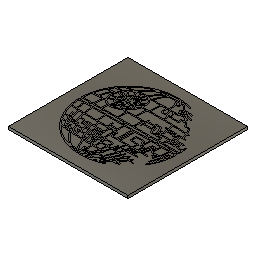
Death Star display v8 (Autodesk Fusion 360 archive; units mm, degrees)
design "Death Star display" references "autodesk 3ax table head yxz"
Autodesk Fusion 360 part; units mm, degrees
(part 1 of 5)
sketch "Sketch1" plane through (0, 0, 0) normal (0, 0, 1) x (1, 0, 0)
  spline S0 degree 3 poles (-1.6299, -34.337) (-1.7839, -34.323) (-2.351, -34.2778) (-2.89, -34.2364) knots 0 0 0 0 1 1 1 1
  spline S1 degree 3 poles (-2.89, -34.2364) (-5.9502, -34.0018) (-9.4769, -33.1887) (-12.4456, -32.0334) knots 0 0 0 0 1 1 1 1
  spline S2 degree 3 poles (-12.4456, -32.0334) (-13.5279, -31.6122) (-13.855, -31.4671) (-15.2108, -30.8071) knots 0 0 0 0 1 1 1 1
  spline S3 degree 3 poles (-15.2108, -30.8071) (-22.0231, -27.4905) (-27.7431, -21.7969) (-31.0912, -15.0001) knots 0 0 0 0 1 1 1 1
  spline S4 degree 3 poles (-31.0912, -15.0001) (-33.1398, -10.8414) (-34.2254, -6.8844) (-34.6063, -2.1874) knots 0 0 0 0 1 1 1 1
  line L0 (-34.6063, -2.1874) -> (-34.7219, -0.7625)
  line L1 (-34.7219, -0.7625) -> (-34.4344, -0.4696)
  line L2 (-34.4344, -0.4696) -> (-34.1469, -0.1767)
  line L3 (-34.1469, -0.1767) -> (-34.1469, 0.483)
  line L4 (-34.1469, 0.483) -> (-34.1469, 1.1428)
  line L5 (-34.1469, 1.1428) -> (-34.4351, 1.4363)
  line L6 (-34.4351, 1.4363) -> (-34.7232, 1.7299)
  line L7 (-34.7232, 1.7299) -> (-34.6057, 3.1541)
  spline S5 degree 3 poles (-34.6057, 3.1541) (-33.9079, 11.6096) (-30.3961, 19.2356) (-24.4881, 25.1245) knots 0 0 0 0 1 1 1 1
  spline S6 degree 3 poles (-24.4881, 25.1245) (-18.2485, 31.3441) (-10.2507, 34.8631) (-1.4199, 35.2745) knots 0 0 0 0 1 1 1 1
  spline S7 degree 3 poles (-1.4199, 35.2745) (2.3869, 35.4519) (6.2534, 34.994) (9.9208, 33.9317) knots 0 0 0 0 1 1 1 1
  spline S8 degree 3 poles (9.9208, 33.9317) (10.9671, 33.6286) (11.0739, 33.5871) (11.2449, 33.416) knots 0 0 0 0 1 1 1 1
  spline S9 degree 3 poles (11.2449, 33.416) (11.3437, 33.3172) (11.3441, 33.2853) (11.2485, 33.1006) knots 0 0 0 0 1 1 1 1
  spline S10 degree 3 poles (11.2485, 33.1006) (11.1766, 32.9614) (11.089, 32.895) (10.9772, 32.895) knots 0 0 0 0 1 1 1 1
  spline S11 degree 3 poles (10.9772, 32.895) (10.8864, 32.895) (10.3281, 33.0339) (9.7364, 33.2037) knots 0 0 0 0 1 1 1 1
  spline S12 degree 3 poles (9.7364, 33.2037) (8.2848, 33.6202) (6.6384, 33.9815) (5.2556, 34.1871) knots 0 0 0 0 1 1 1 1
  spline S13 degree 3 poles (5.2556, 34.1871) (4.2003, 34.3439) (4.1036, 34.3483) (4.0229, 34.2428) knots 0 0 0 0 1 1 1 1
  spline S14 degree 3 poles (4.0229, 34.2428) (3.8864, 34.0642) (3.9187, 33.9997) (4.2949, 33.7001) knots 0 0 0 0 1 1 1 1
  spline S15 degree 3 poles (4.2949, 33.7001) (5.0546, 33.0949) (4.9616, 33.1289) (6.0085, 33.0734) knots 0 0 0 0 1 1 1 1
  spline S16 degree 3 poles (6.0085, 33.0734) (6.537, 33.0454) (7.0379, 32.9965) (7.1215, 32.9647) knots 0 0 0 0 1 1 1 1
  spline S17 degree 3 poles (7.1215, 32.9647) (7.3715, 32.8696) (8.6397, 31.827) (9.4234, 31.0722) knots 0 0 0 0 1 1 1 1
  line L8 (9.4234, 31.0722) -> (10.156, 30.3666)
  line L9 (10.156, 30.3666) -> (11.0184, 30.3026)
  spline S18 degree 3 poles (11.0184, 30.3026) (12.8168, 30.1691) (15.6071, 29.7574) (16.0637, 29.5581) knots 0 0 0 0 1 1 1 1
  spline S19 degree 3 poles (16.0637, 29.5581) (16.3282, 29.4427) (16.3625, 29.3626) (16.2798, 29.0535) knots 0 0 0 0 1 1 1 1
  spline S20 degree 3 poles (16.2798, 29.0535) (16.2375, 28.8956) (16.214, 28.8893) (15.8082, 28.9275) knots 0 0 0 0 1 1 1 1
  spline S21 degree 3 poles (15.8082, 28.9275) (15.5733, 28.9497) (15.1291, 29.0129) (14.8211, 29.0681) knots 0 0 0 0 1 1 1 1
  spline S22 degree 3 poles (14.8211, 29.0681) (13.6561, 29.2768) (13.6729, 29.2766) (13.5839, 29.0812) knots 0 0 0 0 1 1 1 1
  spline S23 degree 3 poles (13.5839, 29.0812) (13.5104, 28.9199) (13.5347, 28.8729) (13.8828, 28.5027) knots 0 0 0 0 1 1 1 1
  spline S24 degree 3 poles (13.8828, 28.5027) (14.0912, 28.2811) (14.3876, 27.9481) (14.5414, 27.7628) knots 0 0 0 0 1 1 1 1
  line L10 (14.5414, 27.7628) -> (14.8211, 27.4259)
  line L11 (14.8211, 27.4259) -> (15.5806, 27.3262)
  spline S25 degree 3 poles (15.5806, 27.3262) (17.4175, 27.0852) (18.6937, 26.7735) (18.9731, 26.4976) knots 0 0 0 0 1 1 1 1
  spline S26 degree 3 poles (18.9731, 26.4976) (19.0983, 26.3741) (19.1239, 26.2944) (19.0866, 26.1456) knots 0 0 0 0 1 1 1 1
  spline S27 degree 3 poles (19.0866, 26.1456) (19.0601, 26.0398) (18.9925, 25.9357) (18.9365, 25.9142) knots 0 0 0 0 1 1 1 1
  spline S28 degree 3 poles (18.9365, 25.9142) (18.8805, 25.8927) (18.4829, 25.9714) (18.053, 26.0889) knots 0 0 0 0 1 1 1 1
  spline S29 degree 3 poles (18.053, 26.0889) (16.8455, 26.4192) (15.9994, 26.5611) (15.8713, 26.4547) knots 0 0 0 0 1 1 1 1
  spline S30 degree 3 poles (15.8713, 26.4547) (15.7138, 26.324) (15.7436, 26.1435) (15.9612, 25.9106) knots 0 0 0 0 1 1 1 1
  spline S31 degree 3 poles (15.9612, 25.9106) (16.1292, 25.7307) (16.2251, 25.6949) (16.6531, 25.6519) knots 0 0 0 0 1 1 1 1
  spline S32 degree 3 poles (16.6531, 25.6519) (17.2658, 25.5904) (17.5932, 25.4158) (17.5357, 25.1814) knots 0 0 0 0 1 1 1 1
  spline S33 degree 3 poles (17.5357, 25.1814) (17.4779, 24.9455) (17.3792, 24.8445) (17.2067, 24.8445) knots 0 0 0 0 1 1 1 1
  spline S34 degree 3 poles (17.2067, 24.8445) (17.0335, 24.8445) (16.8862, 24.7229) (16.8862, 24.5799) knots 0 0 0 0 1 1 1 1
  spline S35 degree 3 poles (16.8862, 24.5799) (16.8862, 24.5267) (16.9924, 24.3204) (17.1221, 24.1213) knots 0 0 0 0 1 1 1 1
  spline S36 degree 3 poles (17.1221, 24.1213) (17.2518, 23.9223) (17.443, 23.6113) (17.5469, 23.4301) knots 0 0 0 0 1 1 1 1
  spline S37 degree 3 poles (17.5469, 23.4301) (17.7574, 23.0631) (17.7742, 23.055) (18.4569, 22.9881) knots 0 0 0 0 1 1 1 1
  spline S38 degree 3 poles (18.4569, 22.9881) (18.724, 22.9619) (19.0145, 22.8933) (19.1025, 22.8357) knots 0 0 0 0 1 1 1 1
  spline S39 degree 3 poles (19.1025, 22.8357) (19.2689, 22.7266) (19.8565, 21.8786) (20.241, 21.1925) knots 0 0 0 0 1 1 1 1
  spline S40 degree 3 poles (20.241, 21.1925) (20.3633, 20.9742) (20.5012, 20.7648) (20.5474, 20.7272) knots 0 0 0 0 1 1 1 1
  spline S41 degree 3 poles (20.5474, 20.7272) (20.5936, 20.6895) (21.2844, 20.6109) (22.0824, 20.5524) knots 0 0 0 0 1 1 1 1
  spline S42 degree 3 poles (22.0824, 20.5524) (23.3363, 20.4606) (23.5611, 20.4264) (23.738, 20.3004) knots 0 0 0 0 1 1 1 1
  spline S43 degree 3 poles (23.738, 20.3004) (23.8876, 20.1939) (24.1714, 19.6967) (24.7902, 18.4568) knots 0 0 0 0 1 1 1 1
  spline S44 degree 3 poles (24.7902, 18.4568) (25.2563, 17.523) (25.6374, 16.7208) (25.6372, 16.674) knots 0 0 0 0 1 1 1 1
  spline S45 degree 3 poles (25.6372, 16.674) (25.6364, 16.5295) (25.857, 16.4643) (26.5118, 16.4154) knots 0 0 0 0 1 1 1 1
  spline S46 degree 3 poles (26.5118, 16.4154) (26.8583, 16.3895) (27.2442, 16.3357) (27.3694, 16.2957) knots 0 0 0 0 1 1 1 1
  spline S47 degree 3 poles (27.3694, 16.2957) (27.5664, 16.2329) (27.5969, 16.1917) (27.5969, 15.9883) knots 0 0 0 0 1 1 1 1
  spline S48 degree 3 poles (27.5969, 15.9883) (27.5969, 15.698) (27.468, 15.6443) (26.8199, 15.6645) knots 0 0 0 0 1 1 1 1
  spline S49 degree 3 poles (26.8199, 15.6645) (26.2136, 15.6833) (26.1253, 15.5947) (26.2847, 15.1273) knots 0 0 0 0 1 1 1 1
  spline S50 degree 3 poles (26.2847, 15.1273) (26.3463, 14.9467) (26.5579, 14.3264) (26.7551, 13.7488) knots 0 0 0 0 1 1 1 1
  spline S51 degree 3 poles (26.7551, 13.7488) (26.9522, 13.1713) (27.1653, 12.6594) (27.2286, 12.6113) knots 0 0 0 0 1 1 1 1
  spline S52 degree 3 poles (27.2286, 12.6113) (27.3005, 12.5565) (27.5755, 12.5238) (27.9625, 12.5238) knots 0 0 0 0 1 1 1 1
  spline S53 degree 3 poles (27.9625, 12.5238) (28.7632, 12.5238) (29.067, 12.4088) (29.067, 12.1058) knots 0 0 0 0 1 1 1 1
  spline S54 degree 3 poles (29.067, 12.1058) (29.067, 11.7499) (28.92, 11.7252) (27.3051, 11.8106) knots 0 0 0 0 1 1 1 1
  spline S55 degree 3 poles (27.3051, 11.8106) (26.0171, 11.8787) (25.8721, 11.875) (25.7564, 11.7703) knots 0 0 0 0 1 1 1 1
  spline S56 degree 3 poles (25.7564, 11.7703) (25.6664, 11.6888) (25.6422, 11.6024) (25.6741, 11.4768) knots 0 0 0 0 1 1 1 1
  spline S57 degree 3 poles (25.6741, 11.4768) (25.8258, 10.8804) (26.1968, 9.1892) (26.1968, 9.094) knots 0 0 0 0 1 1 1 1
  spline S58 degree 3 poles (26.1968, 9.094) (26.1968, 9.0315) (26.2378, 8.9243) (26.2878, 8.8558) knots 0 0 0 0 1 1 1 1
  spline S59 degree 3 poles (26.2878, 8.8558) (26.397, 8.7065) (26.4181, 8.7047) (29.347, 8.5979) knots 0 0 0 0 1 1 1 1
  spline S60 degree 3 poles (29.347, 8.5979) (31.7762, 8.5093) (31.9372, 8.4796) (31.9372, 8.1202) knots 0 0 0 0 1 1 1 1
  spline S61 degree 3 poles (31.9372, 8.1202) (31.9372, 7.8265) (31.6603, 7.7329) (30.9701, 7.7931) knots 0 0 0 0 1 1 1 1
  spline S62 degree 3 poles (30.9701, 7.7931) (30.4875, 7.8352) (30.4115, 7.8254) (30.3047, 7.7074) knots 0 0 0 0 1 1 1 1
  spline S63 degree 3 poles (30.3047, 7.7074) (30.1903, 7.5811) (30.1932, 7.5183) (30.3606, 6.4987) knots 0 0 0 0 1 1 1 1
  spline S64 degree 3 poles (30.3606, 6.4987) (30.4577, 5.9071) (30.5371, 5.3334) (30.5371, 5.2236) knots 0 0 0 0 1 1 1 1
  spline S65 degree 3 poles (30.5371, 5.2236) (30.5371, 4.7238) (30.5851, 4.7101) (32.5383, 4.6524) knots 0 0 0 0 1 1 1 1
  line L12 (32.5383, 4.6524) -> (33.8045, 4.6149)
  line L13 (33.8045, 4.6149) -> (33.8905, 4.7757)
  spline S66 degree 3 poles (33.8905, 4.7757) (33.9606, 4.9066) (33.9499, 5.1007) (33.8326, 5.8222) knots 0 0 0 0 1 1 1 1
  spline S67 degree 3 poles (33.8326, 5.8222) (33.6677, 6.8367) (33.6971, 7.0284) (34.025, 7.0765) knots 0 0 0 0 1 1 1 1
  spline S68 degree 3 poles (34.025, 7.0765) (34.3629, 7.1261) (34.4398, 6.9157) (34.6693, 5.3133) knots 0 0 0 0 1 1 1 1
  spline S69 degree 3 poles (34.6693, 5.3133) (34.7859, 4.4989) (34.9467, 2.6691) (34.9471, 2.1532) knots 0 0 0 0 1 1 1 1
  spline S70 degree 3 poles (34.9471, 2.1532) (34.9473, 1.7163) (34.9311, 1.6686) (34.6759, 1.3598) knots 0 0 0 0 1 1 1 1
  spline S71 degree 3 poles (34.6759, 1.3598) (34.4089, 1.0367) (34.4046, 1.0223) (34.4134, 0.4812) knots 0 0 0 0 1 1 1 1
  spline S72 degree 3 poles (34.4134, 0.4812) (34.4219, -0.0405) (34.4358, -0.0867) (34.6848, -0.4131) knots 0 0 0 0 1 1 1 1
  spline S73 degree 3 poles (34.6848, -0.4131) (34.925, -0.728) (34.9473, -0.7954) (34.9471, -1.2047) knots 0 0 0 0 1 1 1 1
  spline S74 degree 3 poles (34.9471, -1.2047) (34.9465, -1.8462) (34.7588, -3.799) (34.5982, -4.8304) knots 0 0 0 0 1 1 1 1
  spline S75 degree 3 poles (34.5982, -4.8304) (34.0278, -8.4945) (32.9754, -11.7968) (31.3273, -15.0929) knots 0 0 0 0 1 1 1 1
  spline S76 degree 3 poles (31.3273, -15.0929) (30.3393, -17.0691) (30.1369, -17.336) (29.7956, -17.1124) knots 0 0 0 0 1 1 1 1
  spline S77 degree 3 poles (29.7956, -17.1124) (29.6431, -17.0125) (29.6224, -16.9596) (29.6593, -16.763) knots 0 0 0 0 1 1 1 1
  spline S78 degree 3 poles (29.6593, -16.763) (29.6832, -16.6356) (29.815, -16.3337) (29.9521, -16.0922) knots 0 0 0 0 1 1 1 1
  spline S79 degree 3 poles (29.9521, -16.0922) (30.3995, -15.3042) (31.0971, -13.8729) (31.0971, -13.7429) knots 0 0 0 0 1 1 1 1
  spline S80 degree 3 poles (31.0971, -13.7429) (31.0971, -13.5327) (30.9653, -13.4645) (30.6197, -13.4961) knots 0 0 0 0 1 1 1 1
  spline S81 degree 3 poles (30.6197, -13.4961) (30.0164, -13.5513) (29.9895, -13.5672) (29.7731, -13.9958) knots 0 0 0 0 1 1 1 1
  spline S82 degree 3 poles (29.7731, -13.9958) (29.5066, -14.5239) (29.4404, -14.5729) (29.1561, -14.4536) knots 0 0 0 0 1 1 1 1
  spline S83 degree 3 poles (29.1561, -14.4536) (28.9511, -14.3676) (28.9342, -14.3378) (28.9727, -14.1309) knots 0 0 0 0 1 1 1 1
  spline S84 degree 3 poles (28.9727, -14.1309) (28.9961, -14.0055) (29.2122, -13.3988) (29.453, -12.7828) knots 0 0 0 0 1 1 1 1
  spline S85 degree 3 poles (29.453, -12.7828) (29.985, -11.4215) (30.4454, -10.0193) (30.7741, -8.7592) knots 0 0 0 0 1 1 1 1
  spline S86 degree 3 poles (30.7741, -8.7592) (31.0871, -7.5589) (31.0954, -7.5736) (30.1326, -7.62) knots 0 0 0 0 1 1 1 1
  spline S87 degree 3 poles (30.1326, -7.62) (29.6266, -7.6443) (29.423, -7.6822) (29.3388, -7.7676) knots 0 0 0 0 1 1 1 1
  spline S88 degree 3 poles (29.3388, -7.7676) (29.2726, -7.8348) (29.117, -8.377) (28.9642, -9.0726) knots 0 0 0 0 1 1 1 1
  spline S89 degree 3 poles (28.9642, -9.0726) (28.549, -10.9622) (28.4593, -11.1542) (28.0627, -11.0023) knots 0 0 0 0 1 1 1 1
  spline S90 degree 3 poles (28.0627, -11.0023) (27.8758, -10.9308) (27.8653, -10.9055) (27.8924, -10.5944) knots 0 0 0 0 1 1 1 1
  spline S91 degree 3 poles (27.8924, -10.5944) (27.9083, -10.4119) (28.0415, -9.7353) (28.1884, -9.0909) knots 0 0 0 0 1 1 1 1
  spline S92 degree 3 poles (28.1884, -9.0909) (28.4059, -8.1361) (28.4391, -7.8995) (28.3676, -7.8133) knots 0 0 0 0 1 1 1 1
  spline S93 degree 3 poles (28.3676, -7.8133) (28.2583, -7.6816) (27.674, -7.6707) (27.5011, -7.7971) knots 0 0 0 0 1 1 1 1
  spline S94 degree 3 poles (27.5011, -7.7971) (27.4276, -7.8508) (27.328, -8.1099) (27.2522, -8.4446) knots 0 0 0 0 1 1 1 1
  spline S95 degree 3 poles (27.2522, -8.4446) (27.0519, -9.3288) (26.9738, -9.5736) (26.8383, -9.7409) knots 0 0 0 0 1 1 1 1
  spline S96 degree 3 poles (26.8383, -9.7409) (26.7304, -9.8742) (26.681, -9.8874) (26.5067, -9.8297) knots 0 0 0 0 1 1 1 1
  spline S97 degree 3 poles (26.5067, -9.8297) (26.2354, -9.7398) (26.2176, -9.5474) (26.4066, -8.7426) knots 0 0 0 0 1 1 1 1
  spline S98 degree 3 poles (26.4066, -8.7426) (26.4889, -8.3918) (26.5378, -8.0312) (26.5152, -7.9412) knots 0 0 0 0 1 1 1 1
  spline S99 degree 3 poles (26.5152, -7.9412) (26.4743, -7.7779) (26.4711, -7.7775) (25.3255, -7.7775) knots 0 0 0 0 1 1 1 1
  line L14 (25.3255, -7.7775) -> (24.1769, -7.7775)
  line L15 (24.1769, -7.7775) -> (23.9618, -7.5165)
  spline S100 degree 3 poles (23.9618, -7.5165) (23.8435, -7.373) (23.7467, -7.2008) (23.7467, -7.134) knots 0 0 0 0 1 1 1 1
  spline S101 degree 3 poles (23.7467, -7.134) (23.7467, -6.867) (23.0285, -6.7555) (22.8186, -6.9899) knots 0 0 0 0 1 1 1 1
  spline S102 degree 3 poles (22.8186, -6.9899) (22.7547, -7.0613) (22.6474, -7.4785) (22.5614, -7.9898) knots 0 0 0 0 1 1 1 1
  spline S103 degree 3 poles (22.5614, -7.9898) (22.4803, -8.4724) (22.3249, -9.3018) (22.216, -9.833) knots 0 0 0 0 1 1 1 1
  spline S104 degree 3 poles (22.216, -9.833) (21.9451, -11.1548) (21.8426, -11.0705) (23.6417, -11.0042) knots 0 0 0 0 1 1 1 1
  spline S105 degree 3 poles (23.6417, -11.0042) (25.2698, -10.9442) (25.4268, -10.9717) (25.4268, -11.3171) knots 0 0 0 0 1 1 1 1
  spline S106 degree 3 poles (25.4268, -11.3171) (25.4268, -11.4801) (25.3842, -11.5756) (25.2885, -11.6268) knots 0 0 0 0 1 1 1 1
  spline S107 degree 3 poles (25.2885, -11.6268) (25.1384, -11.7072) (22.5954, -11.8346) (21.104, -11.8366) knots 0 0 0 0 1 1 1 1
  spline S108 degree 3 poles (21.104, -11.8366) (20.2707, -11.8376) (20.1622, -11.852) (20.0364, -11.9778) knots 0 0 0 0 1 1 1 1
  spline S109 degree 3 poles (20.0364, -11.9778) (19.9594, -12.0548) (19.8964, -12.1629) (19.8964, -12.218) knots 0 0 0 0 1 1 1 1
  spline S110 degree 3 poles (19.8964, -12.218) (19.8964, -12.3489) (19.354, -14.4146) (19.2646, -14.6244) knots 0 0 0 0 1 1 1 1
  spline S111 degree 3 poles (19.2646, -14.6244) (19.2176, -14.7346) (19.2207, -14.8326) (19.2743, -14.9328) knots 0 0 0 0 1 1 1 1
  spline S112 degree 3 poles (19.2743, -14.9328) (19.3513, -15.0766) (19.3806, -15.0787) (20.7064, -15.0343) knots 0 0 0 0 1 1 1 1
  spline S113 degree 3 poles (20.7064, -15.0343) (22.2673, -14.982) (22.4166, -15.0102) (22.4166, -15.3572) knots 0 0 0 0 1 1 1 1
  spline S114 degree 3 poles (22.4166, -15.3572) (22.4166, -15.5566) (22.384, -15.6013) (22.1891, -15.67) knots 0 0 0 0 1 1 1 1
  spline S115 degree 3 poles (22.1891, -15.67) (21.9751, -15.7454) (20.071, -15.8452) (17.2012, -15.9315) knots 0 0 0 0 1 1 1 1
  spline S116 degree 3 poles (17.2012, -15.9315) (16.5082, -15.9524) (15.4904, -15.9888) (14.9395, -16.0124) knots 0 0 0 0 1 1 1 1
  spline S117 degree 3 poles (14.9395, -16.0124) (13.7776, -16.0622) (13.8181, -16.0365) (13.6328, -16.8431) knots 0 0 0 0 1 1 1 1
  spline S118 degree 3 poles (13.6328, -16.8431) (13.5709, -17.1126) (13.4084, -17.7232) (13.2718, -18.1999) knots 0 0 0 0 1 1 1 1
  spline S119 degree 3 poles (13.2718, -18.1999) (12.9494, -19.3249) (12.9251, -19.2946) (14.2001, -19.3546) knots 0 0 0 0 1 1 1 1
  spline S120 degree 3 poles (14.2001, -19.3546) (14.9341, -19.3892) (15.1353, -19.3786) (15.199, -19.3018) knots 0 0 0 0 1 1 1 1
  spline S121 degree 3 poles (15.199, -19.3018) (15.2428, -19.249) (15.3974, -18.8946) (15.5424, -18.5144) knots 0 0 0 0 1 1 1 1
  spline S122 degree 3 poles (15.5424, -18.5144) (15.8798, -17.6298) (15.9501, -17.5081) (16.1232, -17.5081) knots 0 0 0 0 1 1 1 1
  spline S123 degree 3 poles (16.1232, -17.5081) (16.5865, -17.5081) (16.6391, -17.7921) (16.3262, -18.6046) knots 0 0 0 0 1 1 1 1
  spline S124 degree 3 poles (16.3262, -18.6046) (16.2107, -18.9046) (16.1162, -19.1852) (16.1162, -19.2283) knots 0 0 0 0 1 1 1 1
  spline S125 degree 3 poles (16.1162, -19.2283) (16.1162, -19.4449) (16.371, -19.5217) (17.2488, -19.5698) knots 0 0 0 0 1 1 1 1
  spline S126 degree 3 poles (17.2488, -19.5698) (18.2871, -19.6267) (18.1667, -19.7081) (18.6413, -18.6282) knots 0 0 0 0 1 1 1 1
  spline S127 degree 3 poles (18.6413, -18.6282) (18.802, -18.2624) (18.9969, -17.8936) (19.0743, -17.8087) knots 0 0 0 0 1 1 1 1
  spline S128 degree 3 poles (19.0743, -17.8087) (19.2055, -17.6647) (19.2287, -17.6612) (19.4157, -17.7579) knots 0 0 0 0 1 1 1 1
  spline S129 degree 3 poles (19.4157, -17.7579) (19.693, -17.9013) (19.6812, -18.1981) (19.3714, -18.878) knots 0 0 0 0 1 1 1 1
  spline S130 degree 3 poles (19.3714, -18.878) (19.0989, -19.476) (19.0839, -19.5558) (19.2222, -19.6706) knots 0 0 0 0 1 1 1 1
  spline S131 degree 3 poles (19.2222, -19.6706) (19.3492, -19.776) (20.8787, -19.962) (21.0157, -19.8886) knots 0 0 0 0 1 1 1 1
  spline S132 degree 3 poles (21.0157, -19.8886) (21.0746, -19.8571) (21.2695, -19.5679) (21.4487, -19.246) knots 0 0 0 0 1 1 1 1
  spline S133 degree 3 poles (21.4487, -19.246) (21.628, -18.924) (21.8425, -18.5992) (21.9254, -18.5242) knots 0 0 0 0 1 1 1 1
  spline S134 degree 3 poles (21.9254, -18.5242) (22.0636, -18.3991) (22.0917, -18.3965) (22.2633, -18.4929) knots 0 0 0 0 1 1 1 1
  spline S135 degree 3 poles (22.2633, -18.4929) (22.5344, -18.645) (22.5308, -18.7917) (22.2419, -19.3763) knots 0 0 0 0 1 1 1 1
  spline S136 degree 3 poles (22.2419, -19.3763) (22.0019, -19.8618) (21.9919, -19.9071) (22.0975, -20.0238) knots 0 0 0 0 1 1 1 1
  spline S137 degree 3 poles (22.0975, -20.0238) (22.1651, -20.0985) (22.359, -20.1668) (22.5763, -20.1925) knots 0 0 0 0 1 1 1 1
  spline S138 degree 3 poles (22.5763, -20.1925) (23.2927, -20.2773) (24.4852, -20.5929) (24.6804, -20.7493) knots 0 0 0 0 1 1 1 1
  spline S139 degree 3 poles (24.6804, -20.7493) (24.8574, -20.8912) (24.8662, -20.9211) (24.7927, -21.1308) knots 0 0 0 0 1 1 1 1
  spline S140 degree 3 poles (24.7927, -21.1308) (24.7255, -21.3228) (24.6786, -21.3582) (24.4923, -21.3576) knots 0 0 0 0 1 1 1 1
  spline S141 degree 3 poles (24.4923, -21.3576) (24.371, -21.357) (24.1142, -21.3087) (23.9216, -21.2499) knots 0 0 0 0 1 1 1 1
  spline S142 degree 3 poles (23.9216, -21.2499) (23.4341, -21.1009) (21.6392, -20.791) (21.5088, -20.8333) knots 0 0 0 0 1 1 1 1
  spline S143 degree 3 poles (21.5088, -20.8333) (21.4498, -20.8524) (21.1691, -21.2383) (20.885, -21.6907) knots 0 0 0 0 1 1 1 1
  spline S144 degree 3 poles (20.885, -21.6907) (20.2516, -22.6996) (19.7939, -23.3575) (19.1863, -24.1324) knots 0 0 0 0 1 1 1 1
  spline S145 degree 3 poles (19.1863, -24.1324) (18.852, -24.5587) (18.7317, -24.7655) (18.7585, -24.8679) knots 0 0 0 0 1 1 1 1
  spline S146 degree 3 poles (18.7585, -24.8679) (18.779, -24.9463) (18.8308, -25.0205) (18.8735, -25.0329) knots 0 0 0 0 1 1 1 1
  spline S147 degree 3 poles (18.8735, -25.0329) (20.1001, -25.3867) (20.4228, -25.6622) (20.2083, -26.1724) knots 0 0 0 0 1 1 1 1
  spline S148 degree 3 poles (20.2083, -26.1724) (20.085, -26.4656) (19.6172, -26.6956) (18.776, -26.8766) knots 0 0 0 0 1 1 1 1
  spline S149 degree 3 poles (18.776, -26.8766) (18.185, -27.0038) (16.7415, -27.2387) (16.551, -27.2387) knots 0 0 0 0 1 1 1 1
  spline S150 degree 3 poles (16.551, -27.2387) (16.5113, -27.2387) (16.1688, -27.5252) (15.7899, -27.8754) knots 0 0 0 0 1 1 1 1
  spline S151 degree 3 poles (15.7899, -27.8754) (14.7516, -28.8352) (13.5283, -29.7985) (12.4388, -30.5143) knots 0 0 0 0 1 1 1 1
  spline S152 degree 3 poles (12.4388, -30.5143) (10.9769, -31.4747) (10.9358, -31.5033) (10.9358, -31.5615) knots 0 0 0 0 1 1 1 1
  spline S153 degree 3 poles (10.9358, -31.5615) (10.9358, -31.5911) (10.9962, -31.653) (11.07, -31.6991) knots 0 0 0 0 1 1 1 1
  spline S154 degree 3 poles (11.07, -31.6991) (11.1827, -31.7694) (11.3767, -31.7174) (12.2776, -31.375) knots 0 0 0 0 1 1 1 1
  spline S155 degree 3 poles (12.2776, -31.375) (12.868, -31.1507) (13.5991, -30.8528) (13.9023, -30.713) knots 0 0 0 0 1 1 1 1
  spline S156 degree 3 poles (13.9023, -30.713) (14.6088, -30.3873) (14.8758, -30.3786) (14.9995, -30.6771) knots 0 0 0 0 1 1 1 1
  spline S157 degree 3 poles (14.9995, -30.6771) (15.0829, -30.8785) (15.0768, -30.9059) (14.9205, -31.0315) knots 0 0 0 0 1 1 1 1
  spline S158 degree 3 poles (14.9205, -31.0315) (14.1992, -31.6112) (10.4693, -32.9271) (7.904, -33.5068) knots 0 0 0 0 1 1 1 1
  spline S159 degree 3 poles (7.904, -33.5068) (5.3056, -34.094) (3.3463, -34.3212) (0.6802, -34.3446) knots 0 0 0 0 1 1 1 1
  spline S160 degree 3 poles (0.6802, -34.3446) (-0.4364, -34.3544) (-1.4759, -34.351) (-1.6299, -34.337) knots 0 0 0 0 1 1 1 1
  spline S161 degree 3 poles (0.5866, -33.4262) (0.8687, -33.2307) (1.3308, -32.5888) (1.6567, -31.9396) knots 0 0 0 0 1 1 1 1
  spline S162 degree 3 poles (1.6567, -31.9396) (1.8353, -31.5837) (1.8387, -31.5587) (1.7241, -31.4321) knots 0 0 0 0 1 1 1 1
  spline S163 degree 3 poles (1.7241, -31.4321) (1.613, -31.3094) (1.4898, -31.299) (0.1552, -31.299) knots 0 0 0 0 1 1 1 1
  spline S164 degree 3 poles (0.1552, -31.299) (-1.154, -31.299) (-1.3042, -31.3111) (-1.408, -31.4258) knots 0 0 0 0 1 1 1 1
  spline S165 degree 3 poles (-1.408, -31.4258) (-1.5031, -31.5309) (-1.509, -31.5889) (-1.4423, -31.7656) knots 0 0 0 0 1 1 1 1
  spline S166 degree 3 poles (-1.4423, -31.7656) (-1.3704, -31.956) (-1.3838, -32.0111) (-1.5687, -32.2863) knots 0 0 0 0 1 1 1 1
  line L16 (-1.5687, -32.2863) -> (-1.7754, -32.594)
  line L17 (-1.7754, -32.594) -> (-2.6477, -32.5733)
  spline S167 degree 3 poles (-2.6477, -32.5733) (-3.9188, -32.5432) (-6.0557, -32.4294) (-7.0039, -32.3414) knots 0 0 0 0 1 1 1 1
  spline S168 degree 3 poles (-7.0039, -32.3414) (-7.457, -32.2993) (-7.8744, -32.2829) (-7.9315, -32.3048) knots 0 0 0 0 1 1 1 1
  spline S169 degree 3 poles (-7.9315, -32.3048) (-8.0176, -32.3378) (-8.089, -32.629) (-8.0109, -32.629) knots 0 0 0 0 1 1 1 1
  spline S170 degree 3 poles (-8.0109, -32.629) (-7.9975, -32.629) (-7.6274, -32.7085) (-7.1884, -32.8056) knots 0 0 0 0 1 1 1 1
  spline S171 degree 3 poles (-7.1884, -32.8056) (-5.0974, -33.2682) (-2.7361, -33.5495) (-0.5527, -33.5962) knots 0 0 0 0 1 1 1 1
  spline S172 degree 3 poles (-0.5527, -33.5962) (0.2892, -33.6142) (0.3225, -33.6093) (0.5866, -33.4262) knots 0 0 0 0 1 1 1 1
  spline S173 degree 3 poles (3.6663, -33.3618) (4.4067, -33.2061) (5.5101, -32.8226) (6.2063, -32.479) knots 0 0 0 0 1 1 1 1
  spline S174 degree 3 poles (6.2063, -32.479) (6.7486, -32.2115) (6.8099, -32.1617) (6.7914, -32.004) knots 0 0 0 0 1 1 1 1
  spline S175 degree 3 poles (6.7914, -32.004) (6.7707, -31.8289) (6.7665, -31.8279) (6.1406, -31.8441) knots 0 0 0 0 1 1 1 1
  spline S176 degree 3 poles (6.1406, -31.8441) (5.794, -31.8531) (5.1438, -31.8797) (4.6957, -31.9033) knots 0 0 0 0 1 1 1 1
  line L18 (4.6957, -31.9033) -> (3.8809, -31.9461)
  line L19 (3.8809, -31.9461) -> (3.3447, -32.5718)
  spline S177 degree 3 poles (3.3447, -32.5718) (2.9446, -33.0389) (2.8195, -33.232) (2.8517, -33.3333) knots 0 0 0 0 1 1 1 1
  spline S178 degree 3 poles (2.8517, -33.3333) (2.9037, -33.4971) (3.0059, -33.5007) (3.6663, -33.3618) knots 0 0 0 0 1 1 1 1
  spline S179 degree 3 poles (8.7206, -32.5207) (9.8615, -32.2332) (10.099, -32.0722) (9.8094, -31.7826) knots 0 0 0 0 1 1 1 1
  spline S180 degree 3 poles (9.8094, -31.7826) (9.5788, -31.552) (9.0686, -31.6449) (8.5436, -32.0132) knots 0 0 0 0 1 1 1 1
  spline S181 degree 3 poles (8.5436, -32.0132) (8.1231, -32.3081) (8.1064, -32.3312) (8.1782, -32.5183) knots 0 0 0 0 1 1 1 1
  spline S182 degree 3 poles (8.1782, -32.5183) (8.2298, -32.6529) (8.1965, -32.6527) (8.7206, -32.5207) knots 0 0 0 0 1 1 1 1
  line L20 (8.7206, -32.5207) -> (8.7206, -32.5207)
  spline S183 degree 3 poles (3.3834, -31.2461) (3.7678, -30.6821) (4.5356, -29.2497) (4.8475, -28.5146) knots 0 0 0 0 1 1 1 1
  spline S184 degree 3 poles (4.8475, -28.5146) (4.9953, -28.1663) (4.9974, -28.138) (4.8853, -28.0141) knots 0 0 0 0 1 1 1 1
  spline S185 degree 3 poles (4.8853, -28.0141) (4.7855, -27.9039) (4.6972, -27.8887) (4.3335, -27.9191) knots 0 0 0 0 1 1 1 1
  spline S186 degree 3 poles (4.3335, -27.9191) (4.0953, -27.9391) (3.861, -27.9922) (3.8129, -28.0372) knots 0 0 0 0 1 1 1 1
  spline S187 degree 3 poles (3.8129, -28.0372) (3.7647, -28.0821) (3.6017, -28.5745) (3.4507, -29.1314) knots 0 0 0 0 1 1 1 1
  spline S188 degree 3 poles (3.4507, -29.1314) (3.1892, -30.0957) (2.8076, -31.2578) (2.6629, -31.531) knots 0 0 0 0 1 1 1 1
  spline S189 degree 3 poles (2.6629, -31.531) (2.5812, -31.6851) (2.7126, -31.8754) (2.8789, -31.8438) knots 0 0 0 0 1 1 1 1
  spline S190 degree 3 poles (2.8789, -31.8438) (2.9402, -31.8322) (3.1672, -31.5632) (3.3834, -31.2461) knots 0 0 0 0 1 1 1 1
  spline S191 degree 3 poles (-2.435, -31.649) (-2.3817, -31.5494) (-2.3818, -31.4684) (-2.4352, -31.3684) knots 0 0 0 0 1 1 1 1
  spline S192 degree 3 poles (-2.4352, -31.3684) (-2.5502, -31.1536) (-3.0271, -29.6625) (-3.2099, -28.9464) knots 0 0 0 0 1 1 1 1
  line L21 (-3.2099, -28.9464) -> (-3.3727, -28.3089)
  line L22 (-3.3727, -28.3089) -> (-3.1513, -28.0293)
  line L23 (-3.1513, -28.0293) -> (-2.9299, -27.7498)
  line L24 (-2.9299, -27.7498) -> (-2.2449, -27.7824)
  spline S193 degree 3 poles (-2.2449, -27.7824) (-1.2629, -27.8292) (-1.3055, -27.9189) (-1.4469, -26.103) knots 0 0 0 0 1 1 1 1
  spline S194 degree 3 poles (-1.4469, -26.103) (-1.5311, -25.0223) (-1.5867, -24.6258) (-1.6649, -24.5485) knots 0 0 0 0 1 1 1 1
  spline S195 degree 3 poles (-1.6649, -24.5485) (-1.7535, -24.4608) (-2.177, -24.443) (-4.3853, -24.4343) knots 0 0 0 0 1 1 1 1
  spline S196 degree 3 poles (-4.3853, -24.4343) (-7.4101, -24.4224) (-7.3062, -24.4016) (-7.0921, -24.9771) knots 0 0 0 0 1 1 1 1
  spline S197 degree 3 poles (-7.0921, -24.9771) (-6.0772, -27.7053) (-4.8716, -29.9792) (-3.7209, -31.3355) knots 0 0 0 0 1 1 1 1
  line L25 (-3.7209, -31.3355) -> (-3.3362, -31.789)
  line L26 (-3.3362, -31.789) -> (-2.923, -31.789)
  spline S198 degree 3 poles (-2.923, -31.789) (-2.5815, -31.789) (-2.4969, -31.7647) (-2.4349, -31.649) knots 0 0 0 0 1 1 1 1
  line L27 (-2.4349, -31.649) -> (-2.435, -31.649)
  spline S199 degree 3 poles (-4.7428, -31.5747) (-4.6767, -31.4511) (-4.725, -31.3435) (-5.0806, -30.8222) knots 0 0 0 0 1 1 1 1
  spline S200 degree 3 poles (-5.0806, -30.8222) (-6.0754, -29.3639) (-7.3421, -26.7506) (-7.9239, -24.9565) knots 0 0 0 0 1 1 1 1
  spline S201 degree 3 poles (-7.9239, -24.9565) (-8.1247, -24.3372) (-7.8894, -24.3916) (-10.9055, -24.2676) knots 0 0 0 0 1 1 1 1
  spline S202 degree 3 poles (-10.9055, -24.2676) (-13.1644, -24.1747) (-14.6122, -24.1002) (-16.0779, -24.0013) knots 0 0 0 0 1 1 1 1
  spline S203 degree 3 poles (-16.0779, -24.0013) (-16.2502, -23.9897) (-16.3408, -24.0242) (-16.4094, -24.1276) knots 0 0 0 0 1 1 1 1
  spline S204 degree 3 poles (-16.4094, -24.1276) (-16.4954, -24.2571) (-16.4624, -24.3225) (-16.0383, -24.8617) knots 0 0 0 0 1 1 1 1
  spline S205 degree 3 poles (-16.0383, -24.8617) (-14.5307, -26.7783) (-12.5618, -28.6748) (-10.756, -29.9496) knots 0 0 0 0 1 1 1 1
  spline S206 degree 3 poles (-10.756, -29.9496) (-10.1749, -30.3598) (-9.0016, -31.0902) (-8.5573, -31.3183) knots 0 0 0 0 1 1 1 1
  spline S207 degree 3 poles (-8.5573, -31.3183) (-8.3296, -31.4352) (-7.4699, -31.5488) (-6.1102, -31.6417) knots 0 0 0 0 1 1 1 1
  spline S208 degree 3 poles (-6.1102, -31.6417) (-4.7819, -31.7324) (-4.8285, -31.7347) (-4.7428, -31.5747) knots 0 0 0 0 1 1 1 1
  spline S209 degree 3 poles (-11.0374, -30.9338) (-10.9643, -30.7973) (-10.978, -30.7616) (-11.1512, -30.6363) knots 0 0 0 0 1 1 1 1
  spline S210 degree 3 poles (-11.1512, -30.6363) (-13.3038, -29.0789) (-15.455, -26.9497) (-17.0946, -24.7535) knots 0 0 0 0 1 1 1 1
  spline S211 degree 3 poles (-17.0946, -24.7535) (-17.3532, -24.407) (-17.6069, -24.0719) (-17.6581, -24.0087) knots 0 0 0 0 1 1 1 1
  spline S212 degree 3 poles (-17.6581, -24.0087) (-17.716, -23.9375) (-17.9068, -23.8782) (-18.1612, -23.8524) knots 0 0 0 0 1 1 1 1
  spline S213 degree 3 poles (-18.1612, -23.8524) (-18.3866, -23.8296) (-19.0908, -23.7596) (-19.726, -23.697) knots 0 0 0 0 1 1 1 1
  spline S214 degree 3 poles (-19.726, -23.697) (-20.3613, -23.6343) (-21.5427, -23.4889) (-22.3512, -23.3738) knots 0 0 0 0 1 1 1 1
  spline S215 degree 3 poles (-22.3512, -23.3738) (-24.1806, -23.1135) (-24.068, -23.1202) (-24.1612, -23.265) knots 0 0 0 0 1 1 1 1
  spline S216 degree 3 poles (-24.1612, -23.265) (-24.2273, -23.3677) (-24.1636, -23.4639) (-23.7503, -23.8842) knots 0 0 0 0 1 1 1 1
  spline S217 degree 3 poles (-23.7503, -23.8842) (-21.5232, -26.1502) (-18.3509, -28.4123) (-15.1507, -30.0166) knots 0 0 0 0 1 1 1 1
  spline S218 degree 3 poles (-15.1507, -30.0166) (-14.2623, -30.462) (-14.1802, -30.4882) (-12.7606, -30.7798) knots 0 0 0 0 1 1 1 1
  spline S219 degree 3 poles (-12.7606, -30.7798) (-11.9521, -30.9458) (-11.2523, -31.0833) (-11.2055, -31.0853) knots 0 0 0 0 1 1 1 1
  spline S220 degree 3 poles (-11.2055, -31.0853) (-11.1587, -31.0874) (-11.0831, -31.0191) (-11.0374, -30.9338) knots 0 0 0 0 1 1 1 1
  spline S221 degree 3 poles (7.807, -30.5424) (8.4998, -29.9566) (9.3374, -29.1303) (9.8943, -28.4833) knots 0 0 0 0 1 1 1 1
  spline S222 degree 3 poles (9.8943, -28.4833) (10.2631, -28.0548) (10.2963, -27.991) (10.218, -27.8606) knots 0 0 0 0 1 1 1 1
  spline S223 degree 3 poles (10.218, -27.8606) (10.1369, -27.7255) (10.0864, -27.7181) (9.5008, -27.7556) knots 0 0 0 0 1 1 1 1
  spline S224 degree 3 poles (9.5008, -27.7556) (9.1542, -27.7777) (8.2407, -27.8161) (7.4706, -27.8409) knots 0 0 0 0 1 1 1 1
  spline S225 degree 3 poles (7.4706, -27.8409) (6.7006, -27.8657) (6.0339, -27.9153) (5.9891, -27.9509) knots 0 0 0 0 1 1 1 1
  spline S226 degree 3 poles (5.9891, -27.9509) (5.9443, -27.9866) (5.7749, -28.3214) (5.6126, -28.6948) knots 0 0 0 0 1 1 1 1
  spline S227 degree 3 poles (5.6126, -28.6948) (5.4503, -29.0683) (5.1452, -29.7133) (4.9345, -30.1283) knots 0 0 0 0 1 1 1 1
  spline S228 degree 3 poles (4.9345, -30.1283) (4.413, -31.1557) (4.3747, -31.1215) (5.9865, -31.0685) knots 0 0 0 0 1 1 1 1
  line L28 (5.9865, -31.0685) -> (7.2334, -31.0275)
  line L29 (7.2334, -31.0275) -> (7.807, -30.5424)
  spline S229 degree 3 poles (2.1634, -30.4739) (2.2091, -30.4448) (2.2781, -30.3382) (2.3166, -30.2369) knots 0 0 0 0 1 1 1 1
  spline S230 degree 3 poles (2.3166, -30.2369) (2.3726, -30.0895) (2.3619, -30.0303) (2.2629, -29.9408) knots 0 0 0 0 1 1 1 1
  spline S231 degree 3 poles (2.2629, -29.9408) (2.1557, -29.8437) (1.874, -29.8289) (0.143, -29.8289) knots 0 0 0 0 1 1 1 1
  spline S232 degree 3 poles (0.143, -29.8289) (-1.7355, -29.8289) (-1.8604, -29.8368) (-1.9747, -29.963) knots 0 0 0 0 1 1 1 1
  spline S233 degree 3 poles (-1.9747, -29.963) (-2.0765, -30.0755) (-2.0822, -30.1236) (-2.0101, -30.2606) knots 0 0 0 0 1 1 1 1
  spline S234 degree 3 poles (-2.0101, -30.2606) (-1.9627, -30.3504) (-1.8893, -30.447) (-1.847, -30.4753) knots 0 0 0 0 1 1 1 1
  spline S235 degree 3 poles (-1.847, -30.4753) (-1.7451, -30.5434) (2.0563, -30.542) (2.1634, -30.474) knots 0 0 0 0 1 1 1 1
  line L30 (2.1634, -30.474) -> (2.1634, -30.4739)
  spline S236 degree 3 poles (11.6878, -28.6866) (12.1207, -28.2945) (12.4751, -27.9404) (12.4754, -27.8996) knots 0 0 0 0 1 1 1 1
  spline S237 degree 3 poles (12.4754, -27.8996) (12.4756, -27.8589) (12.4366, -27.7725) (12.3884, -27.7077) knots 0 0 0 0 1 1 1 1
  spline S238 degree 3 poles (12.3884, -27.7077) (12.3175, -27.6122) (12.2312, -27.5982) (11.9332, -27.6341) knots 0 0 0 0 1 1 1 1
  spline S239 degree 3 poles (11.9332, -27.6341) (11.5696, -27.6778) (11.5596, -27.6855) (11.0508, -28.316) knots 0 0 0 0 1 1 1 1
  spline S240 degree 3 poles (11.0508, -28.316) (10.7678, -28.6668) (10.3229, -29.1833) (10.0623, -29.4637) knots 0 0 0 0 1 1 1 1
  spline S241 degree 3 poles (10.0623, -29.4637) (9.6068, -29.9537) (9.593, -29.9788) (9.7091, -30.1071) knots 0 0 0 0 1 1 1 1
  spline S242 degree 3 poles (9.7091, -30.1071) (9.8268, -30.237) (9.8442, -30.2294) (10.3654, -29.82) knots 0 0 0 0 1 1 1 1
  spline S243 degree 3 poles (10.3654, -29.82) (10.6599, -29.5887) (11.255, -29.0787) (11.6878, -28.6866) knots 0 0 0 0 1 1 1 1
  spline S244 degree 3 poles (12.9074, -29.2587) (13.5315, -28.7988) (14.65, -27.8848) (14.7287, -27.7705) knots 0 0 0 0 1 1 1 1
  spline S245 degree 3 poles (14.7287, -27.7705) (14.7549, -27.7324) (14.7459, -27.6444) (14.7087, -27.575) knots 0 0 0 0 1 1 1 1
  spline S246 degree 3 poles (14.7087, -27.575) (14.6291, -27.4263) (14.201, -27.405) (13.981, -27.5389) knots 0 0 0 0 1 1 1 1
  spline S247 degree 3 poles (13.981, -27.5389) (13.904, -27.5857) (13.4383, -28.0361) (12.9461, -28.5396) knots 0 0 0 0 1 1 1 1
  spline S248 degree 3 poles (12.9461, -28.5396) (12.2929, -29.2079) (12.0633, -29.4867) (12.0961, -29.572) knots 0 0 0 0 1 1 1 1
  spline S249 degree 3 poles (12.0961, -29.572) (12.1684, -29.7605) (12.2906, -29.7133) (12.9074, -29.2587) knots 0 0 0 0 1 1 1 1
  spline S250 degree 3 poles (2.6602, -28.9713) (2.7539, -28.8574) (3.0967, -27.4519) (3.4063, -25.9122) knots 0 0 0 0 1 1 1 1
  spline S251 degree 3 poles (3.4063, -25.9122) (3.6382, -24.7585) (3.6453, -24.6834) (3.5329, -24.5593) knots 0 0 0 0 1 1 1 1
  spline S252 degree 3 poles (3.5329, -24.5593) (3.4202, -24.4347) (3.3099, -24.4299) (1.4199, -24.4679) knots 0 0 0 0 1 1 1 1
  spline S253 degree 3 poles (1.4199, -24.4679) (-0.0878, -24.4982) (-0.5966, -24.5303) (-0.666, -24.5997) knots 0 0 0 0 1 1 1 1
  spline S254 degree 3 poles (-0.666, -24.5997) (-0.7562, -24.6899) (-0.7347, -25.3746) (-0.5753, -27.4837) knots 0 0 0 0 1 1 1 1
  spline S255 degree 3 poles (-0.5753, -27.4837) (-0.5339, -28.0306) (-0.5378, -28.0495) (-0.7411, -28.2888) knots 0 0 0 0 1 1 1 1
  spline S256 degree 3 poles (-0.7411, -28.2888) (-0.9491, -28.5335) (-0.9501, -28.5338) (-1.5924, -28.5471) knots 0 0 0 0 1 1 1 1
  spline S257 degree 3 poles (-1.5924, -28.5471) (-2.2157, -28.5599) (-2.435, -28.6279) (-2.435, -28.8084) knots 0 0 0 0 1 1 1 1
  spline S258 degree 3 poles (-2.435, -28.8084) (-2.435, -29.0447) (-2.2884, -29.0588) (0.1606, -29.0588) knots 0 0 0 0 1 1 1 1
  spline S259 degree 3 poles (0.1606, -29.0588) (2.0176, -29.0588) (2.6051, -29.0383) (2.6602, -28.9713) knots 0 0 0 0 1 1 1 1
  spline S260 degree 3 poles (5.3522, -27.0564) (5.4924, -27.0142) (6.2004, -24.8946) (6.1628, -24.6299) knots 0 0 0 0 1 1 1 1
  spline S261 degree 3 poles (6.1628, -24.6299) (6.1415, -24.4802) (6.1075, -24.4727) (5.3634, -24.4538) knots 0 0 0 0 1 1 1 1
  spline S262 degree 3 poles (5.3634, -24.4538) (4.7956, -24.4394) (4.567, -24.4583) (4.5149, -24.5238) knots 0 0 0 0 1 1 1 1
  spline S263 degree 3 poles (4.5149, -24.5238) (4.4756, -24.5732) (4.3429, -25.1286) (4.2199, -25.7581) knots 0 0 0 0 1 1 1 1
  spline S264 degree 3 poles (4.2199, -25.7581) (4.0065, -26.8505) (4.0019, -26.9087) (4.1186, -27.0377) knots 0 0 0 0 1 1 1 1
  spline S265 degree 3 poles (4.1186, -27.0377) (4.2249, -27.1552) (4.3053, -27.1676) (4.7357, -27.1329) knots 0 0 0 0 1 1 1 1
  spline S266 degree 3 poles (4.7357, -27.1329) (5.0078, -27.111) (5.2853, -27.0766) (5.3522, -27.0564) knots 0 0 0 0 1 1 1 1
  spline S267 degree 3 poles (9.9908, -26.9599) (10.5683, -26.928) (11.0881, -26.8828) (11.1459, -26.8594) knots 0 0 0 0 1 1 1 1
  spline S268 degree 3 poles (11.1459, -26.8594) (11.2734, -26.8078) (12.1959, -25.451) (12.1959, -25.3152) knots 0 0 0 0 1 1 1 1
  spline S269 degree 3 poles (12.1959, -25.3152) (12.1959, -25.1059) (12.0048, -25.0278) (11.453, -25.0119) knots 0 0 0 0 1 1 1 1
  spline S270 degree 3 poles (11.453, -25.0119) (11.1493, -25.0031) (10.8635, -25.0207) (10.8178, -25.0511) knots 0 0 0 0 1 1 1 1
  spline S271 degree 3 poles (10.8178, -25.0511) (10.7721, -25.0815) (10.641, -25.2947) (10.5266, -25.525) knots 0 0 0 0 1 1 1 1
  spline S272 degree 3 poles (10.5266, -25.525) (10.4121, -25.7552) (10.2381, -26.0188) (10.1399, -26.1108) knots 0 0 0 0 1 1 1 1
  spline S273 degree 3 poles (10.1399, -26.1108) (9.9782, -26.2621) (9.9412, -26.2696) (9.7485, -26.1898) knots 0 0 0 0 1 1 1 1
  spline S274 degree 3 poles (9.7485, -26.1898) (9.4625, -26.0713) (9.4736, -25.9241) (9.8231, -25.2049) knots 0 0 0 0 1 1 1 1
  spline S275 degree 3 poles (9.8231, -25.2049) (10.5254, -23.7597) (11.1916, -22.1546) (11.7159, -20.6442) knots 0 0 0 0 1 1 1 1
  spline S276 degree 3 poles (11.7159, -20.6442) (11.9396, -19.9999) (11.9227, -19.9892) (10.6068, -19.9346) knots 0 0 0 0 1 1 1 1
  spline S277 degree 3 poles (10.6068, -19.9346) (8.9205, -19.8646) (8.3034, -19.8753) (8.2212, -19.9758) knots 0 0 0 0 1 1 1 1
  spline S278 degree 3 poles (8.2212, -19.9758) (8.1818, -20.0239) (8.0819, -20.3783) (7.999, -20.7633) knots 0 0 0 0 1 1 1 1
  spline S279 degree 3 poles (7.999, -20.7633) (7.615, -22.5484) (7.0845, -24.5558) (6.6337, -25.9301) knots 0 0 0 0 1 1 1 1
  spline S280 degree 3 poles (6.6337, -25.9301) (6.3619, -26.759) (6.3428, -26.8879) (6.4731, -27.0182) knots 0 0 0 0 1 1 1 1
  spline S281 degree 3 poles (6.4731, -27.0182) (6.5638, -27.1089) (7.6063, -27.0916) (9.9908, -26.9599) knots 0 0 0 0 1 1 1 1
  spline S282 degree 3 poles (13.793, -26.4846) (14.7408, -25.4238) (14.7555, -25.2568) (13.9077, -25.18) knots 0 0 0 0 1 1 1 1
  spline S283 degree 3 poles (13.9077, -25.18) (13.5421, -25.1469) (13.3431, -25.157) (13.2766, -25.2122) knots 0 0 0 0 1 1 1 1
  spline S284 degree 3 poles (13.2766, -25.2122) (13.2232, -25.2565) (13.0036, -25.5716) (12.7885, -25.9125) knots 0 0 0 0 1 1 1 1
  spline S285 degree 3 poles (12.7885, -25.9125) (12.4473, -26.4533) (12.4079, -26.5514) (12.4787, -26.6838) knots 0 0 0 0 1 1 1 1
  spline S286 degree 3 poles (12.4787, -26.6838) (12.5542, -26.8248) (12.5948, -26.8322) (13.0604, -26.7898) knots 0 0 0 0 1 1 1 1
  spline S287 degree 3 poles (13.0604, -26.7898) (13.5249, -26.7476) (13.5778, -26.7255) (13.793, -26.4846) knots 0 0 0 0 1 1 1 1
  spline S288 degree 3 poles (15.893, -26.5387) (16.0155, -26.5387) (16.1856, -26.4206) (16.4433, -26.1567) knots 0 0 0 0 1 1 1 1
  spline S289 degree 3 poles (16.4433, -26.1567) (16.8462, -25.744) (16.8604, -25.7132) (16.7287, -25.5409) knots 0 0 0 0 1 1 1 1
  spline S290 degree 3 poles (16.7287, -25.5409) (16.6661, -25.459) (16.5041, -25.4204) (16.1584, -25.405) knots 0 0 0 0 1 1 1 1
  line L31 (16.1584, -25.405) -> (15.6755, -25.3836)
  line L32 (15.6755, -25.3836) -> (15.3285, -25.8222)
  spline S291 degree 3 poles (15.3285, -25.8222) (15.0444, -26.1812) (14.9898, -26.294) (15.0274, -26.4437) knots 0 0 0 0 1 1 1 1
  spline S292 degree 3 poles (15.0274, -26.4437) (15.0708, -26.6166) (15.091, -26.6243) (15.3945, -26.5827) knots 0 0 0 0 1 1 1 1
  spline S293 degree 3 poles (15.3945, -26.5827) (15.5712, -26.5585) (15.7955, -26.5387) (15.893, -26.5387) knots 0 0 0 0 1 1 1 1
  spline S294 degree 3 poles (18.5798, -26.1453) (18.6799, -26.0834) (18.6399, -25.785) (18.5256, -25.7411) knots 0 0 0 0 1 1 1 1
  spline S295 degree 3 poles (18.5256, -25.7411) (18.2888, -25.6502) (17.8879, -25.6987) (17.7665, -25.8328) knots 0 0 0 0 1 1 1 1
  spline S296 degree 3 poles (17.7665, -25.8328) (17.667, -25.9428) (17.6599, -25.9947) (17.7275, -26.1209) knots 0 0 0 0 1 1 1 1
  spline S297 degree 3 poles (17.7275, -26.1209) (17.8017, -26.2595) (17.8455, -26.2702) (18.1666, -26.2276) knots 0 0 0 0 1 1 1 1
  spline S298 degree 3 poles (18.1666, -26.2276) (18.3628, -26.2015) (18.5487, -26.1645) (18.5798, -26.1453) knots 0 0 0 0 1 1 1 1
  spline S299 degree 3 poles (17.6913, -24.735) (17.9396, -24.5526) (19.1299, -22.9742) (19.8564, -21.864) knots 0 0 0 0 1 1 1 1
  spline S300 degree 3 poles (19.8564, -21.864) (20.6621, -20.633) (20.6719, -20.6622) (19.4064, -20.5212) knots 0 0 0 0 1 1 1 1
  spline S301 degree 3 poles (19.4064, -20.5212) (18.6143, -20.433) (18.699, -20.3691) (18.0646, -21.5333) knots 0 0 0 0 1 1 1 1
  spline S302 degree 3 poles (18.0646, -21.5333) (17.562, -22.4556) (16.7851, -23.7595) (16.5591, -24.0601) knots 0 0 0 0 1 1 1 1
  spline S303 degree 3 poles (16.5591, -24.0601) (16.2657, -24.4502) (16.3735, -24.6602) (16.8997, -24.7239) knots 0 0 0 0 1 1 1 1
  spline S304 degree 3 poles (16.8997, -24.7239) (17.446, -24.79) (17.6132, -24.7923) (17.6913, -24.735) knots 0 0 0 0 1 1 1 1
  spline S305 degree 3 poles (15.7518, -23.896) (16.272, -23.1175) (16.9136, -22.0556) (17.3368, -21.2727) knots 0 0 0 0 1 1 1 1
  spline S306 degree 3 poles (17.3368, -21.2727) (17.8193, -20.3801) (17.7991, -20.3553) (16.5184, -20.2681) knots 0 0 0 0 1 1 1 1
  spline S307 degree 3 poles (16.5184, -20.2681) (16.0383, -20.2354) (15.8063, -20.2459) (15.737, -20.3035) knots 0 0 0 0 1 1 1 1
  spline S308 degree 3 poles (15.737, -20.3035) (15.6827, -20.3485) (15.5074, -20.6909) (15.3474, -21.0643) knots 0 0 0 0 1 1 1 1
  spline S309 degree 3 poles (15.3474, -21.0643) (15.1874, -21.4378) (14.7854, -22.2903) (14.4541, -22.9588) knots 0 0 0 0 1 1 1 1
  spline S310 degree 3 poles (14.4541, -22.9588) (13.9855, -23.9043) (13.8676, -24.1997) (13.9235, -24.2889) knots 0 0 0 0 1 1 1 1
  spline S311 degree 3 poles (13.9235, -24.2889) (13.9961, -24.4048) (14.3679, -24.4761) (15.0118, -24.4975) knots 0 0 0 0 1 1 1 1
  line L33 (15.0118, -24.4975) -> (15.3425, -24.5085)
  line L34 (15.3425, -24.5085) -> (15.7518, -23.896)
  spline S312 degree 3 poles (12.9148, -24.176) (13.0629, -24.0119) (14.0585, -22.0689) (14.474, -21.1332) knots 0 0 0 0 1 1 1 1
  spline S313 degree 3 poles (14.474, -21.1332) (14.8599, -20.264) (14.8467, -20.1986) (14.2737, -20.1401) knots 0 0 0 0 1 1 1 1
  spline S314 degree 3 poles (14.2737, -20.1401) (13.2534, -20.036) (12.8813, -20.0429) (12.7559, -20.1683) knots 0 0 0 0 1 1 1 1
  spline S315 degree 3 poles (12.7559, -20.1683) (12.6885, -20.2358) (12.5302, -20.602) (12.4043, -20.9822) knots 0 0 0 0 1 1 1 1
  spline S316 degree 3 poles (12.4043, -20.9822) (12.2784, -21.3623) (11.9738, -22.1774) (11.7275, -22.7934) knots 0 0 0 0 1 1 1 1
  spline S317 degree 3 poles (11.7275, -22.7934) (11.2208, -24.0608) (11.21, -24.2048) (11.6187, -24.2475) knots 0 0 0 0 1 1 1 1
  spline S318 degree 3 poles (11.6187, -24.2475) (12.347, -24.3238) (12.8043, -24.2985) (12.9148, -24.176) knots 0 0 0 0 1 1 1 1
  spline S319 degree 3 poles (-0.3288, -23.6205) (-0.2432, -23.5349) (-0.2333, -18.3517) (-0.3186, -18.2664) knots 0 0 0 0 1 1 1 1
  spline S320 degree 3 poles (-0.3186, -18.2664) (-0.4228, -18.1622) (-2.4441, -18.1873) (-2.5509, -18.2941) knots 0 0 0 0 1 1 1 1
  spline S321 degree 3 poles (-2.5509, -18.2941) (-2.628, -18.3712) (-2.6197, -18.677) (-2.5016, -20.1001) knots 0 0 0 0 1 1 1 1
  spline S322 degree 3 poles (-2.5016, -20.1001) (-2.265, -22.9506) (-2.1889, -23.5406) (-2.0439, -23.6466) knots 0 0 0 0 1 1 1 1
  spline S323 degree 3 poles (-2.0439, -23.6466) (-1.8949, -23.7555) (-0.4418, -23.7334) (-0.3288, -23.6205) knots 0 0 0 0 1 1 1 1
  spline S324 degree 3 poles (3.767, -23.5749) (3.8497, -23.4869) (3.9294, -23.0212) (4.1735, -21.1988) knots 0 0 0 0 1 1 1 1
  spline S325 degree 3 poles (4.1735, -21.1988) (4.3087, -20.1893) (4.3173, -20.0049) (4.2342, -19.8863) knots 0 0 0 0 1 1 1 1
  spline S326 degree 3 poles (4.2342, -19.8863) (4.1424, -19.7553) (4.0499, -19.7482) (2.4166, -19.7482) knots 0 0 0 0 1 1 1 1
  spline S327 degree 3 poles (2.4166, -19.7482) (0.8597, -19.7482) (0.6868, -19.7599) (0.6026, -19.8707) knots 0 0 0 0 1 1 1 1
  spline S328 degree 3 poles (0.6026, -19.8707) (0.5312, -19.9649) (0.5091, -20.4014) (0.5074, -21.7569) knots 0 0 0 0 1 1 1 1
  spline S329 degree 3 poles (0.5074, -21.7569) (0.5053, -23.5021) (0.5069, -23.5217) (0.6611, -23.6297) knots 0 0 0 0 1 1 1 1
  spline S330 degree 3 poles (0.6611, -23.6297) (0.7949, -23.7234) (1.0199, -23.733) (2.2537, -23.6976) knots 0 0 0 0 1 1 1 1
  spline S331 degree 3 poles (2.2537, -23.6976) (3.2054, -23.6702) (3.7162, -23.6288) (3.767, -23.5749) knots 0 0 0 0 1 1 1 1
  spline S332 degree 3 poles (-4.4006, -23.5387) (-4.3519, -23.4477) (-4.381, -23.0765) (-4.498, -22.2961) knots 0 0 0 0 1 1 1 1
  spline S333 degree 3 poles (-4.498, -22.2961) (-4.8923, -19.6666) (-4.888, -19.4682) (-4.4373, -19.4682) knots 0 0 0 0 1 1 1 1
  spline S334 degree 3 poles (-4.4373, -19.4682) (-4.1377, -19.4682) (-4.0919, -19.585) (-3.9423, -20.7283) knots 0 0 0 0 1 1 1 1
  spline S335 degree 3 poles (-3.9423, -20.7283) (-3.7461, -22.2278) (-3.5349, -23.4931) (-3.4663, -23.581) knots 0 0 0 0 1 1 1 1
  spline S336 degree 3 poles (-3.4663, -23.581) (-3.3725, -23.701) (-3.1707, -23.6909) (-3.0627, -23.5607) knots 0 0 0 0 1 1 1 1
  spline S337 degree 3 poles (-3.0627, -23.5607) (-2.99, -23.473) (-2.995, -23.2219) (-3.0896, -22.2131) knots 0 0 0 0 1 1 1 1
  spline S338 degree 3 poles (-3.0896, -22.2131) (-3.1535, -21.5312) (-3.2534, -20.3748) (-3.3115, -19.6432) knots 0 0 0 0 1 1 1 1
  spline S339 degree 3 poles (-3.3115, -19.6432) (-3.3973, -18.5635) (-3.4393, -18.2967) (-3.5345, -18.2256) knots 0 0 0 0 1 1 1 1
  spline S340 degree 3 poles (-3.5345, -18.2256) (-3.7155, -18.0907) (-5.6096, -18.1038) (-5.7233, -18.2409) knots 0 0 0 0 1 1 1 1
  spline S341 degree 3 poles (-5.7233, -18.2409) (-5.7906, -18.3219) (-5.7852, -18.4908) (-5.6979, -19.0423) knots 0 0 0 0 1 1 1 1
  spline S342 degree 3 poles (-5.6979, -19.0423) (-5.5445, -20.0105) (-5.6097, -20.232) (-6.0497, -20.2373) knots 0 0 0 0 1 1 1 1
  spline S343 degree 3 poles (-6.0497, -20.2373) (-6.2172, -20.2394) (-6.3593, -19.8653) (-6.4672, -19.1383) knots 0 0 0 0 1 1 1 1
  spline S344 degree 3 poles (-6.4672, -19.1383) (-6.5288, -18.7229) (-6.6064, -18.3324) (-6.6395, -18.2704) knots 0 0 0 0 1 1 1 1
  spline S345 degree 3 poles (-6.6395, -18.2704) (-6.6893, -18.1772) (-6.8797, -18.1513) (-7.7351, -18.1211) knots 0 0 0 0 1 1 1 1
  spline S346 degree 3 poles (-7.7351, -18.1211) (-8.4143, -18.0972) (-8.8021, -18.1102) (-8.8627, -18.1589) knots 0 0 0 0 1 1 1 1
  spline S347 degree 3 poles (-8.8627, -18.1589) (-8.9141, -18.2003) (-8.9485, -18.3441) (-8.9404, -18.4832) knots 0 0 0 0 1 1 1 1
  spline S348 degree 3 poles (-8.9404, -18.4832) (-8.909, -19.0224) (-8.9339, -19.1005) (-9.1634, -19.1805) knots 0 0 0 0 1 1 1 1
  spline S349 degree 3 poles (-9.1634, -19.1805) (-9.4309, -19.2737) (-9.4527, -19.2611) (-9.5954, -18.9291) knots 0 0 0 0 1 1 1 1
  spline S350 degree 3 poles (-9.5954, -18.9291) (-9.7901, -18.4758) (-10.391, -15.261) (-10.6658, -13.2028) knots 0 0 0 0 1 1 1 1
  spline S351 degree 3 poles (-10.6658, -13.2028) (-10.7393, -12.6526) (-10.8288, -12.2443) (-10.8923, -12.1703) knots 0 0 0 0 1 1 1 1
  spline S352 degree 3 poles (-10.8923, -12.1703) (-10.9847, -12.0623) (-11.1416, -12.0477) (-12.209, -12.0477) knots 0 0 0 0 1 1 1 1
  spline S353 degree 3 poles (-12.209, -12.0477) (-13.2921, -12.0477) (-13.4275, -12.0608) (-13.4845, -12.1703) knots 0 0 0 0 1 1 1 1
  spline S354 degree 3 poles (-13.4845, -12.1703) (-13.549, -12.2942) (-13.0884, -14.7775) (-12.9392, -15.1104) knots 0 0 0 0 1 1 1 1
  spline S355 degree 3 poles (-12.9392, -15.1104) (-12.8768, -15.2497) (-12.8137, -15.2691) (-12.3946, -15.2779) knots 0 0 0 0 1 1 1 1
  spline S356 degree 3 poles (-12.3946, -15.2779) (-12.1339, -15.2833) (-11.8573, -15.2912) (-11.78, -15.2953) knots 0 0 0 0 1 1 1 1
  spline S357 degree 3 poles (-11.78, -15.2953) (-11.7027, -15.2995) (-11.5359, -15.3836) (-11.4094, -15.4822) knots 0 0 0 0 1 1 1 1
  spline S358 degree 3 poles (-11.4094, -15.4822) (-11.1918, -15.6516) (-11.1647, -15.7259) (-10.9095, -16.8472) knots 0 0 0 0 1 1 1 1
  spline S359 degree 3 poles (-10.9095, -16.8472) (-10.4619, -18.8145) (-9.839, -21.0757) (-9.6716, -21.3408) knots 0 0 0 0 1 1 1 1
  spline S360 degree 3 poles (-9.6716, -21.3408) (-9.5769, -21.4908) (-9.5294, -21.4983) (-8.6723, -21.4983) knots 0 0 0 0 1 1 1 1
  spline S361 degree 3 poles (-8.6723, -21.4983) (-7.5218, -21.4983) (-7.5424, -21.5181) (-7.7365, -20.6024) knots 0 0 0 0 1 1 1 1
  spline S362 degree 3 poles (-7.7365, -20.6024) (-7.903, -19.8169) (-7.8824, -19.4999) (-7.6608, -19.4405) knots 0 0 0 0 1 1 1 1
  spline S363 degree 3 poles (-7.6608, -19.4405) (-7.2356, -19.3264) (-7.2015, -19.3859) (-6.9107, -20.7497) knots 0 0 0 0 1 1 1 1
  spline S364 degree 3 poles (-6.9107, -20.7497) (-6.5768, -22.3157) (-6.2837, -23.4134) (-6.1641, -23.5459) knots 0 0 0 0 1 1 1 1
  spline S365 degree 3 poles (-6.1641, -23.5459) (-6.0712, -23.6489) (-5.927, -23.6685) (-5.2618, -23.6685) knots 0 0 0 0 1 1 1 1
  spline S366 degree 3 poles (-5.2618, -23.6685) (-4.5625, -23.6685) (-4.4619, -23.6533) (-4.4006, -23.5387) knots 0 0 0 0 1 1 1 1
  spline S367 degree 3 poles (6.4743, -23.546) (6.5879, -23.42) (7.0002, -21.811) (7.3325, -20.1971) knots 0 0 0 0 1 1 1 1
  spline S368 degree 3 poles (7.3325, -20.1971) (7.3491, -20.1167) (7.3237, -19.9976) (7.2761, -19.9325) knots 0 0 0 0 1 1 1 1
  spline S369 degree 3 poles (7.2761, -19.9325) (7.2005, -19.8292) (7.0612, -19.8167) (6.1766, -19.8337) knots 0 0 0 0 1 1 1 1
  line L35 (6.1766, -19.8337) -> (5.1637, -19.8532)
  line L36 (5.1637, -19.8532) -> (5.1155, -20.0282)
  spline S370 degree 3 poles (5.1155, -20.0282) (5.0891, -20.1245) (4.9689, -20.9387) (4.8485, -21.8376) knots 0 0 0 0 1 1 1 1
  spline S371 degree 3 poles (4.8485, -21.8376) (4.68, -23.0952) (4.6483, -23.4946) (4.7111, -23.5702) knots 0 0 0 0 1 1 1 1